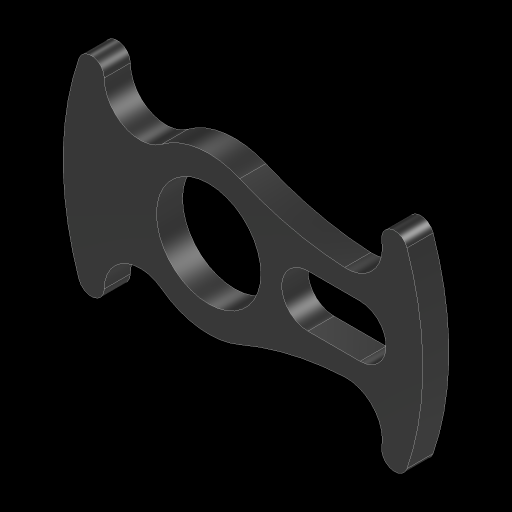
# Autodesk Inventor part: ShufflerFoot
Saved by Autodesk Inventor 2023 (Build 270158000, 158)
## iProperties
Created: 2022-03-05
Part Number: ShufflerFoot
Material: Custom TPU
Document SubType Name: Modeling
Designer: tandu
Density: 1.21 g/cm^3
Appearance: Glossy - Black
Mass: 1.65075 g
Surface Area: 19.1152 cm^2
Volume: 1.75612 cm^3
Author: tandu
Autodesk Inventor part; units mm, degrees
ref_plane "YZ Plane" through (0, 0, 0) normal (1, 0, 0) x (0, 1, 0)
ref_plane "XZ Plane" through (0, 0, 0) normal (0, 1, 0) x (-1, 0, 0)
ref_plane "XY Plane" through (0, 0, 0) normal (0, 0, 1) x (1, 0, 0)
sketch "Sketch1" plane through (0, 0, 0) normal (0, 0, 1) x (1, 0, 0)
  circle A0 centre (0, 0) radius 6.35
  line L0 (18.415, 0) -> (12.065, 0) construction
  line L1 (18.415, 3.175) -> (12.065, 3.175)
  line L2 (12.065, -3.175) -> (18.415, -3.175)
  arc A1 (18.415, -3.175) -> (18.415, 3.175) centre (18.415, 0) ccw
  arc A2 (12.065, 3.175) -> (12.065, -3.175) centre (12.065, 0) ccw
  circle A3 centre (0, 0) radius 9.525
  line L3 (18.415, -5.715) -> (12.065, -5.715)
  arc A4 (12.065, 5.715) -> (12.065, -5.715) centre (12.065, 0) ccw
  line L4 (12.065, 5.715) -> (18.415, 5.715)
  arc A5 (18.415, -5.715) -> (18.415, 5.715) centre (18.415, 0) ccw
  line L5 (-9.525, 0) -> (-15.875, 0) construction
  line L6 (-15.875, -12.7) -> (-15.875, 12.7) construction
  line L7 (-14.2875, 11.1125) -> (-14.2875, -11.1125) construction
  line L8 (-15.875, 11.1125) -> (-15.875, -11.1125)
  line L9 (-12.7, -11.1125) -> (-12.7, 11.1125) construction
  arc A6 (-12.7, 11.1125) -> (-15.875, 11.1125) centre (-14.2875, 11.1125) ccw
  arc A7 (-15.875, -11.1125) -> (-12.7, -11.1125) centre (-14.2875, -11.1125) ccw
  arc A8 (-12.7, 11.1125) -> (-5.715, 7.62) centre (-8.3344, 11.1125) ccw
  arc A9 (-5.715, -7.62) -> (-12.7, -11.1125) centre (-8.3344, -11.1125) ccw
  arc A10 (18.415, -5.715) -> (3.7796, -8.743) centre (18.415, -42.5979) ccw
  arc A11 (3.7796, 8.743) -> (18.415, 5.715) centre (18.415, 42.5979) ccw
  arc A12 (-15.7906, 11.6233) -> (-15.7906, -11.6233) centre (18.415, 0) ccw
  line L10 (0, 0) -> (0, 6.35) construction
  arc A13 (24.13, -11.6233) -> (24.13, 11.6233) centre (-10.0756, 0) ccw
  line L11 (24.13, 11.6233) -> (24.13, -11.6233) construction
  circle A14 centre (22.6269, 11.1125) radius 1.5875 construction
  circle A15 centre (22.6269, -11.1125) radius 1.5875 construction
  arc A16 (21.0615, -10.8486) -> (16.534, -5.763) centre (16.7566, -10.1229) ccw
  arc A17 (16.534, 5.763) -> (21.0615, 10.8486) centre (16.7566, 10.1229) ccw
  arc A18 (24.13, 11.6233) -> (21.0615, 10.8486) centre (22.6269, 11.1125) ccw
  arc A19 (21.0615, -10.8486) -> (24.13, -11.6233) centre (22.6269, -11.1125) ccw
  point P0 (15.24, 0)
  point P1 (-14.2875, 0)
  point P2 (-14.2875, -12.7)
  point P3 (24.13, 0)
  dimension "d0" = 12.7
  dimension "d1" = 6.35
  dimension "d3" = 3.175
  dimension "d4" = 2.54
  dimension "d5" = 6.35
  dimension "d6" = 25.4
  dimension "d7" = 3.175
  dimension "d11" = 6.35
  dimension "d12" = 15.24
  constraints: 47 point on circle, 28 end point, 26 tangent, 19 centre point, 7 equal radius, 4 horizontal alignment, 4 midpoint, 4 vertical, 3 parallel, 2 coincident, 2 horizontal, 2 point on line, 2 vertical alignment, 5 other
  measures "d1" diameter of A2
  measures "d4" distance between parallel lines of L2 L3
  measures "d5" distance of L5.end L5.start
  measures "d6" distance of L6.start L6.end
  measures "d7" diameter of A7
  measures "d11" distance of L0.end L0.start
  measures "d12" distance of point (15.24, 0) point (0, 0)
extrude "Extrusion1" add sketch "Sketch1" along normal blind 3.175 contours A4 A3 | A4 A3 A2 | A4 L4 A5 L3 A3 A2 L2 A1 L1 | A3 A11 L4 A4 | A4 L3 A10 A3 | A3 A9 A7 L8 A6 A8 | A17 A18 A13 A19 A16 A10 A5 A11 | A6 L8 A7 A12
equation "\"d0\" = CamSize1"
equation "\"d1\" = TopStandoffDiameter"
equation "\"d11\" = 2 * Offset1"
equation "\"d12\" = TopStandoffOffset"
equation "\"TopStandoffOffset1\" = 25.4"
equation "\"CamSize1\" = 12.7"
equation "\"TopStandoffDiameter\" = 6.35"
equation "\"Offset1\" = 3.175"
equation "\"TopStandoffOffset\" = 15.24"
body "Solid1"
